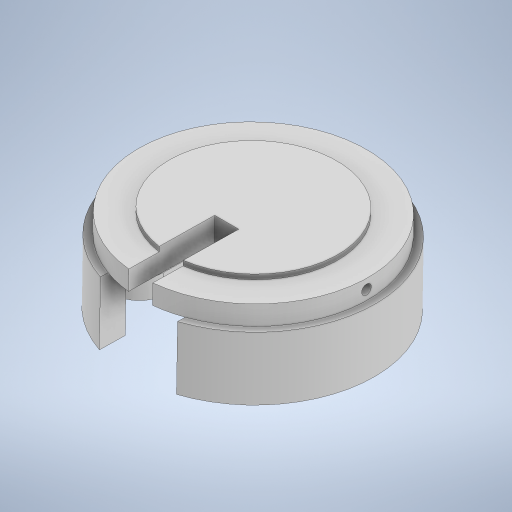
# Autodesk Inventor part: PiezoMount
Saved by Autodesk Inventor 2023 (Build 270158000, 158)
## iProperties
Created: 2023-02-27
Part Number: PiezoMount
Material: Generic
Document SubType Name: Modeling
Designer: maste
Density: 1 g/cm^3
Appearance: Default
Author: maste
Autodesk Inventor part; units mm, degrees
ref_plane "YZ Plane" through (0, 0, 0) normal (1, 0, 0) x (0, 1, 0)
ref_plane "XZ Plane" through (0, 0, 0) normal (0, 1, 0) x (-1, 0, 0)
ref_plane "XY Plane" through (0, 0, 0) normal (0, 0, 1) x (1, 0, 0)
sketch "Sketch1" plane through (0, 0, 0) normal (0, 0, 1) x (1, 0, 0)
  circle A0 centre (0, 0) radius 25
  dimension "d2" = 50
  constraints: 1 centre point, 1 coincident
  measures "d2" diameter of A0
extrude "piezo surface" add sketch "Sketch1" along normal blind 1
sketch "Sketch4" plane through (0, 0, 0) normal (0, 0, -1) x (-1, 0, 0)
  circle A0 centre (0, 0) radius 25 projected
extrude "Depth extension to surface" add sketch "Sketch4" along normal blind 6
sketch "Sketch2" plane through (0, 0, 1) normal (0, 0, 1) x (1, 0, 0)
  circle A0 centre (0, 0) radius 17.95
  circle A1 centre (0, 0) radius 18.75
  line L0 (0, 0) -> (18.75, 0)
  arc A2 (18.75, 0) -> (16.238, 9.375) centre (0, 0) ccw
  line L1 (0, 0) -> (16.238, 9.375) construction
  line L2 (0, 0) -> (18.75, 0) construction
  line L3 (16.238, 9.375) -> (15.5452, 8.975)
  line L4 (0, 0) -> (0, 18.75)
  line L5 (0, 0) -> (0, -18.75)
  line L6 (0, 0) -> (-18.75, 0)
  line L7 (0, 0) -> (-16.238, -9.375)
  line L8 (0, 0) -> (-9.375, 16.238)
  line L9 (0, 0) -> (9.375, -16.238)
  point P0 (17.95, 0)
  point P1 (8.975, -15.5452)
  point P2 (0, -17.95)
  point P3 (-15.5452, -8.975)
  point P4 (-17.95, 0)
  point P5 (-8.975, 15.5452)
  point P6 (0, 17.95)
  dimension "d3" = 35.9
  dimension "d4" = 37.5
  dimension "d5" = 30
  constraints: 20 end point, 4 point on line, 3 coincident, 2 perpendicular, 2 point on circle, 1 centre point, 1 horizontal, 1 vertical, 12 other
  measures "d5" angle of L2 L1
sketch "Sketch3" plane through (0, 0, 1) normal (0, 0, 1) x (1, 0, 0)
  line L0 (0, 0) -> (8.975, -15.5452)
  arc A0 (17.95, 0) -> (15.5452, 8.975) centre (0, 0) ccw projected
  line L1 (0, 0) -> (17.95, 0)
  arc A1 (0, -17.95) -> (8.975, -15.5452) centre (0, 0) ccw projected
  line L2 (8.975, -15.5452) -> (17.95, 0)
  line L3 (13.4625, -7.7726) -> (0, 0)
  line L4 (13.4625, -7.7726) -> (4.8022, -2.7726)
  line L5 (13.4625, -7.7726) -> (4.8022, -2.7726)
  line L6 (13.4625, -7.7726) -> (4.8022, -2.7726)
  line L7 (4.8022, -2.7726) -> (6.0522, -0.6075)
  line L8 (6.0522, -0.6075) -> (14.7125, -5.6075)
  line L9 (14.7125, -5.6075) -> (13.4625, -7.7726)
  line L10 (13.4625, -7.7726) -> (4.8022, -2.7726)
  line L11 (4.8022, -2.7726) -> (3.5522, -4.9376)
  line L12 (3.5522, -4.9376) -> (12.2125, -9.9376)
  line L13 (12.2125, -9.9376) -> (13.4625, -7.7726)
  line L14 (12.2125, -9.9376) -> (14.7125, -5.6075)
  line L15 (14.7125, -5.6075) -> (16.4446, -6.6075)
  line L16 (16.4446, -6.6075) -> (13.9446, -10.9376)
  line L17 (13.9446, -10.9376) -> (12.2125, -9.9376)
  line L18 (-4.802, 2.7724) -> (-3.552, 4.9375)
  line L19 (-3.552, 4.9375) -> (-13.9443, 10.9375)
  line L20 (-4.802, 2.7724) -> (-6.052, 0.6074)
  line L21 (-6.052, 0.6074) -> (-16.4443, 6.6074)
  line L22 (-16.4443, 6.6074) -> (-22.0734, 9.8574)
  line L23 (-22.0734, 9.8574) -> (-19.5734, 14.1875)
  line L24 (-19.5734, 14.1875) -> (-13.9443, 10.9375)
  line L25 (-5.5448, 2.5) -> (-17.5448, 2.5)
  line L26 (-5.5448, 0) -> (-5.5448, 2.5)
  line L27 (-5.5448, 0) -> (-5.5448, -2.5)
  line L28 (-5.5448, -2.5) -> (-17.5448, -2.5)
  line L29 (-17.5448, -2.5) -> (-24.0448, -2.5)
  line L30 (-24.0448, -2.5) -> (-24.0448, 2.5)
  line L31 (-24.0448, 2.5) -> (-17.5448, 2.5)
  point P0 (14.7125, -5.6075)
  point P1 (12.2125, -9.9376)
  point P2 (12.2125, -9.9376)
  dimension "d37" = 10
  dimension "d38" = 2.5
  dimension "d39" = 2.5
  dimension "d40" = 2
  dimension "d49" = 10
  dimension "d69" = 30
  dimension "d71" = 18.5
  dimension "d72" = 5
  constraints: 64 end point, 7 parallel, 4 collinear, 3 perpendicular, 1 midpoint, 1 point on line, 15 other
  measures "d37" distance of L3.start L4.end
  measures "d38" distance of L4.end L7.end
  measures "d39" distance of L11.end L4.end
  measures "d40" distance of L8.end L15.end
  measures "d49" distance between parallel lines of L11 L13
  measures "d71" distance between parallel lines of L30 L27
  measures "d72" distance between parallel lines of L25 L28
extrude "Microphone Wire Hole" cut sketch "Sketch3" against normal blind 14 contours L26 L27 L28 L29 L30 L31 L25 L21 L20 | L20 L21 L25 L26
sketch "Sketch5" plane through (0, 0, -6) normal (0, 0, -1) x (-1, 0, 0)
  line L0 (16, -16) -> (-16, -16)
  line L1 (-16, -16) -> (-16, 16)
  line L2 (-16, 16) -> (16, 16)
  line L3 (16, 16) -> (16, -16)
  line L4 (16, -16) -> (-16, 16) construction
  line L5 (-16, -16) -> (16, 16) construction
  circle A0 centre (0, 0) radius 20
  point P0 (-12, -16)
  point P1 (12, -16)
  point P2 (-16, 12)
  point P3 (-16, -12)
  point P4 (16, 12)
  point P5 (16, -12)
  point P6 (12, 16)
  point P7 (-12, 16)
  dimension "d18" = 32
  dimension "d19" = 32
  dimension "d54" = 40
  constraints: 12 end point, 2 midpoint, 2 parallel, 1 centre point, 1 coincident, 1 horizontal, 1 perpendicular
  measures "d18" distance of L0.start L0.end
  measures "d19" distance of L0.end L1.end
  measures "d54" diameter of A0
extrude "Circuit chamber" cut sketch "Sketch5" against normal blind 3
sketch "Sketch6" plane through (-16, -16, -6) normal (1, 0, 0) x (0, 0, -1)
  line L0 (0, 4) -> (0, 0) projected
  line L1 (0, 32) -> (-3, 32) projected
  line L2 (-3, 32) -> (-3, 28) projected
  line L3 (0, 0) -> (-3, 0) projected
  line L4 (-3, 4) -> (-3, 0) projected
  line L5 (0, 32) -> (0, 28) projected
  line L6 (0, 4) -> (-3, 4) projected
  line L7 (0, -9) -> (0, 41) projected
  line L8 (-7, 41) -> (-7, -9) projected
  line L9 (-3, 32) -> (-3, 28) projected
  line L10 (-3, 32) -> (-3, 32) projected
  line L11 (-3, 28) -> (-3, 32) projected
  line L12 (-3, 4) -> (-3, 28) projected
  line L13 (-3, 0) -> (-3, 4) projected
  line L14 (-3, 0) -> (-3, 0) projected
  line L15 (-3, 4) -> (-3, 0) projected
  line L16 (-3, 13.5) -> (-3, 4) projected
  line L17 (0, -9) -> (0, 41) projected
  line L18 (0, 13.5) -> (0, 4) projected
  line L19 (0, 4) -> (0, 0) projected
  line L20 (0, 0) -> (0, 0) projected
  line L21 (0, 0) -> (0, 4) projected
  line L22 (0, 4) -> (0, 28) projected
  line L23 (0, 28) -> (0, 32) projected
  line L24 (0, 32) -> (0, 32) projected
  line L25 (0, 32) -> (0, 28) projected
  line L26 (-7, 16) -> (0, 16)
  line L27 (0, 16) -> (-3, 16)
  line L28 (-3, 16) -> (-3, 24)
  line L29 (-3, 24) -> (0, 24)
  line L30 (0, 24) -> (0, 16)
  line L31 (0, 16) -> (-3, 16)
  line L32 (-3, 16) -> (-3, 8)
  line L33 (-3, 8) -> (0, 8)
  line L34 (0, 8) -> (0, 16)
  line L35 (0, 28) -> (0, 18.5) projected
  line L36 (0, 18.5) -> (0, 13.5) projected
  line L37 (-3, 18.5) -> (-3, 13.5) projected
  line L38 (-3, 28) -> (-3, 18.5) projected
  line L39 (0, 28) -> (-3, 28) projected
  point P0 (-3, 4)
  point P1 (-3, 8)
  point P2 (0, 8)
  point P3 (-3, 16)
  dimension "d65" = 8
  dimension "d66" = 8
  constraints: 18 end point, 4 parallel, 2 horizontal, 2 midpoint, 2 perpendicular, 2 point on line
  measures "d65" distance of L27.end L28.end
  measures "d66" distance of L32.end L31.end
extrude "port vent" cut sketch "Sketch6" against normal blind 30 contours L33 L12 L26 L7 | L26 L12 L29 L7
sketch "Sketch7" plane through (0, 0, -6) normal (0, 0, -1) x (-1, 0, 0)
  line L0 (0, 0) -> (0, -17.5)
  line L1 (0, 0) -> (0, 17.5)
  dimension "d25" = 17.5
  dimension "d26" = 17.5
  constraints: 4 end point, 2 coincident, 2 vertical
  measures "d25" distance of L0.start L0.end
  measures "d26" distance of L0.start L1.end
hole "screw holes" at (0, 17.5, -6) at (0, -17.5, -6) direction (0, 0, 1) diameter 3.7 depth 4 tip angle 118
sketch "Sketch8" plane through (0, 0, -6) normal (0, 0, -1) x (-1, 0, 0)
  circle A0 centre (0, 0) radius 22.75
  line L0 (21.4137, 11) -> (22.4499, 11) projected
  line L1 (22.4499, 11) -> (19.9139, 11)
  arc A1 (23.6854, 8) -> (23.6854, -8) centre (0, 0) ccw projected
  line L2 (24.6779, -4) -> (22.3956, -4)
  circle A2 centre (0, 0) radius 25 projected
  arc A3 (-16, 12) -> (-16, -12) centre (0, 0) ccw projected
  arc A4 (-12, -16) -> (12, -16) centre (0, 0) ccw projected
  point P0 (12.5, 7.5)
  point P1 (15.0629, 9)
  point P2 (19.2094, 16)
  point P3 (19.2094, -16)
  point P4 (19.9139, 11)
  point P5 (16.7033, 11)
  point P6 (24.6779, 4)
  point P7 (21.9317, -12)
  dimension "d34" = 45.5
  constraints: 4 end point, 2 point on circle, 1 centre point, 1 coincident, 1 horizontal, 1 parallel, 1 other
  measures "d34" diameter of A0
sketch "Sketch9" plane through (0, 0, 0) normal (0, 1, 0) x (-1, 0, 0)
  line L0 (16, -3) -> (-16, -3) projected
  line L1 (0, -3) -> (0, -1)
  circle A0 centre (0, -1) radius 1
  point P0 (0, 0)
  dimension "d41" = 2
  dimension "d42" = 2
  constraints: 2 end point, 1 centre point, 1 coincident, 1 midpoint, 1 vertical
  measures "d41" distance of L1.start L1.end
  measures "d42" diameter of A0
extrude "lock hole" cut sketch "Sketch9" along normal mid plane 100
sketch "Sketch10" plane through (0, 0, -6) normal (0, 0, -1) x (-1, 0, 0)
  arc A0 (23.6854, 8) -> (23.6854, -8) centre (0, 0) ccw projected
  arc A1 (16, -12) -> (18.3303, -8) centre (0, 0) ccw projected
  line L0 (16, -16) -> (12, -16) projected
  arc A2 (-12, -16) -> (12, -16) centre (0, 0) ccw projected
  line L1 (-12, -16) -> (-16, -16) projected
  line L2 (-16, -16) -> (-16, -12) projected
  arc A3 (-16, 12) -> (-16, -12) centre (0, 0) ccw projected
  line L3 (-16, 12) -> (-16, 16) projected
  line L4 (-16, 16) -> (-12, 16) projected
  arc A4 (12, 16) -> (-12, 16) centre (0, 0) ccw projected
  line L5 (12, 16) -> (16, 16) projected
  line L6 (16, 16) -> (16, 12) projected
  line L7 (18.3303, 8) -> (23.6854, 8) projected
  line L8 (23.6854, -8) -> (18.3303, -8) projected
  line L9 (16, -12) -> (16, -16) projected
  arc A5 (18.3303, 8) -> (16, 12) centre (0, 0) ccw projected
extrude "Base Extension" add sketch "Sketch10" along normal blind 10
sketch "Sketch13" plane through (0, 0, 1) normal (0, 0, 1) x (1, 0, 0)
  circle A0 centre (0, 0) radius 25
  circle A1 centre (0, 0) radius 23.5
  dimension "d55" = 47
  dimension "d59" = 50
  constraints: 2 centre point, 2 coincident
  measures "d55" diameter of A1
  measures "d59" diameter of A0
extrude "Rim for flush with diaphragm lock" cut sketch "Sketch13" against normal blind 4
sketch "Sketch14" plane through (-16, 12.1244, -3) normal (1, 0, 0) x (0, 0, -1)
  line L0 (13, -4.1244) -> (13, -20.1244) projected
  line L1 (0, 11.3756) -> (-4, 11.3756) projected
  line L2 (-4, 11.3756) -> (-4, -35.6244) projected
  line L3 (0, -4.1244) -> (0, -20.1244) projected
  line L4 (0, -20.1244) -> (13, -20.1244) projected
  line L5 (13, -4.1244) -> (0, -4.1244) projected
  point P0 (-3, -12.1244)
  point P1 (-4, -2.6061)
  point P2 (-4, 1.724)
sketch "Sketch16" plane through (0, 0, 1) normal (0, 0, 1) x (1, 0, 0)
  circle A0 centre (0, 0) radius 17.25
  arc A1 (-23.3666, -2.5) -> (-23.3666, 2.5) centre (0, 0) ccw projected
  line L0 (-23.3666, 2.5) -> (-5.5448, 2.5) projected
  line L1 (-5.5448, 2.5) -> (-5.5448, -2.5) projected
  line L2 (-5.5448, -2.5) -> (-23.3666, -2.5) projected
  point P0 (-17.0679, -2.5)
  point P1 (-17.0679, 2.5)
  dimension "d73" = 34.5
  constraints: 1 centre point, 1 coincident
  measures "d73" diameter of A0
extrude "Extrusion11" add sketch "Sketch16" along normal blind 1 contours A0 L2 L1 L0 picked at (2.0535, 0)
sketch "Sketch17" plane through (0, 0, -16) normal (0, 0, -1) x (-1, 0, 0)
  arc A0 (12, 16) -> (-12, 16) centre (0, 0) ccw projected
  line L0 (12, 16) -> (-12, 16)
  line L1 (-12, 20.5) -> (12, 20.5)
  line L2 (12, 20.5) -> (12, 11.5)
  line L3 (12, 11.5) -> (-12, 11.5)
  line L4 (-12, 11.5) -> (-12, 20.5)
  line L5 (-12, 20.5) -> (12, 11.5) construction
  line L6 (12, 20.5) -> (-12, 11.5) construction
  arc A1 (-16, 12) -> (-16, -12) centre (0, 0) ccw projected
  line L7 (0, 0) -> (-20, 0)
  line L8 (-12, -20.5) -> (12, -20.5)
  line L9 (12, -20.5) -> (12, -11.5)
  line L10 (12, -11.5) -> (-12, -11.5)
  line L11 (-12, -11.5) -> (-12, -20.5)
  point P0 (0, 16)
  dimension "d76" = 9
  constraints: 24 end point, 4 symmetric about line, 3 midpoint, 2 parallel, 1 horizontal, 1 perpendicular, 1 point on circle
  measures "d76" distance of L1.end L2.end
extrude "Extrusion12" add sketch "Sketch17" against normal blind 4
fillet "Fillet1" radius 5 4 edges at (-12, -11.5, -14) (12, -11.5, -14) (12, 11.5, -14) (-12, 11.5, -14)
sketch "Sketch18" plane through (0, 0, -16) normal (0, 0, -1) x (-1, 0, 0)
  circle A0 centre (0, -17.5) radius 1.85 projected
  circle A1 centre (0, 17.5) radius 1.85 projected
  arc A2 (23.6854, 8) -> (23.6854, -8) centre (0, 0) ccw projected
  dimension "d87" = 17.5
  dimension "d88" = 17.5
  dimension "d92" = 3.7
  measures "d87" distance of A2.centre A1.centre
  measures "d88" distance of point (0, 0) A0.centre
  measures "d92" diameter of A0
extrude "Extrusion13" cut sketch "Sketch18" against normal blind 4
sketch "Sketch19" plane through (0, 0, -12) normal (0, 0, 1) x (1, 0, 0)
  circle A0 centre (0, 17.5) radius 1.85 projected
  arc A1 (-12, 16) -> (-7.0251, 11.5) centre (-7.0251, 16.5) ccw projected
  line L0 (-7.0251, 11.5) -> (7.0251, 11.5) projected
  arc A2 (7.0251, 11.5) -> (12, 16) centre (7.0251, 16.5) ccw projected
  arc A3 (12, 16) -> (-12, 16) centre (0, 0) ccw projected
  line L1 (-1.2512, 20.6061) -> (2.0643, 20.1366)
  circle A4 centre (0, -17.5) radius 1.85 projected
  arc A5 (12, -16) -> (7.0251, -11.5) centre (7.0251, -16.5) ccw projected
  line L2 (7.0251, -11.5) -> (-7.0251, -11.5) projected
  arc A6 (-7.0251, -11.5) -> (-12, -16) centre (-7.0251, -16.5) ccw projected
  arc A7 (-12, -16) -> (12, -16) centre (0, 0) ccw projected
  circle A8 centre (0, -17.5) radius 1.85 projected
  line L3 (3.5161, -17.7003) -> (1.5846, -20.6452)
  line L4 (1.5846, -20.6452) -> (-1.9315, -20.4449)
  line L5 (-1.9315, -20.4449) -> (-3.5161, -17.2997)
  line L6 (-3.5161, -17.2997) -> (-1.5846, -14.3548)
  line L7 (-1.5846, -14.3548) -> (1.9315, -14.5551)
  line L8 (1.9315, -14.5551) -> (3.5161, -17.7003)
  line L9 (1.7609, 20.55) -> (3.5218, 17.5)
  line L10 (3.5218, 17.5) -> (1.7609, 14.45)
  line L11 (1.7609, 14.45) -> (-1.7609, 14.45)
  line L12 (-1.7609, 14.45) -> (-3.5218, 17.5)
  line L13 (-3.5218, 17.5) -> (-1.7609, 20.55)
  line L14 (-1.7609, 20.55) -> (1.7609, 20.55)
  point P0 (-2.2178, -19.8766)
  point P1 (2.0788, -19.8917)
  dimension "d83" = 6.1
  dimension "d86" = 6.1
  constraints: 26 end point, 3 coincident, 28 other
  measures "d83" distance between parallel lines of L6 L3
  measures "d86" distance between parallel lines of L12 L9
extrude "Extrusion14" cut sketch "Sketch19" against normal blind 1 contours A0 | L13 L14 L1 L9 A3 | A3 L9 L10 L11 L12 L13 | L1 L14 L9 | L3 L4 L5 A7 | A7 L5 L6 L7 L8 L3
sketch "Sketch20" plane through (0, 0, -3) normal (0, 0, -1) x (-1, 0, 0)
  circle A0 centre (0, 17.5) radius 1.85 projected
  line L0 (-1.7609, 14.45) -> (1.7609, 14.45) projected
  line L1 (-3.5218, 17.5) -> (-1.7609, 14.45) projected
  line L2 (-1.7609, 20.55) -> (-3.5218, 17.5) projected
  line L3 (1.7609, 20.55) -> (-1.7609, 20.55) projected
  line L4 (3.5218, 17.5) -> (1.7609, 20.55) projected
  line L5 (1.7609, 14.45) -> (3.5218, 17.5) projected
  line L6 (1.5846, -14.3548) -> (-1.9315, -14.5551) projected
  line L7 (3.5161, -17.2997) -> (1.5846, -14.3548) projected
  line L8 (1.9315, -20.4449) -> (3.5161, -17.2997) projected
  line L9 (-3.5161, -17.7003) -> (-1.5846, -20.6452) projected
  line L10 (-1.9315, -14.5551) -> (-3.5161, -17.7003) projected
  circle A1 centre (0, -17.5) radius 1.85 projected
  line L11 (-1.5846, -20.6452) -> (1.9315, -20.4449) projected
  point P0 (0, 0)
  dimension "d91" = 6.1
  measures "d91" distance between parallel lines of L9 L7
extrude "Extrusion15" cut sketch "Sketch20" along normal blind 11 contours L1 L2 L3 L4 L5 L0 | L7 L8 L11 L9 L10 L6 | A1
body "Solid1"
